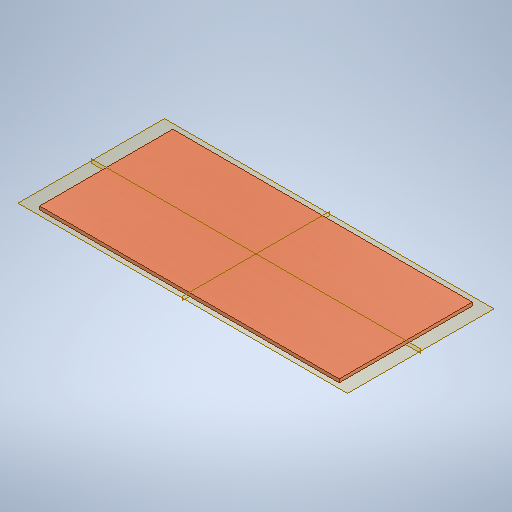
# Autodesk Inventor part: Peça apenas para Exercício
Saved by Autodesk Inventor 2025.2 (Build 292293000, 293)
## iProperties
Created: 2025-04-07
Part Number: Peça apenas para Exercício
Material: Madeira (Nogueira)
Document SubType Name: Modeling
Designer: kenay
Density: 0.55 g/cm^3
Appearance: Nogueira - Natural polido
Author: kenay
Autodesk Inventor part; units mm, degrees
sketch "Esboço1" plane through (0, 0, 0) normal (0, 1, 0) x (-1, 0, 0)
  line L0 (-900, 400) -> (900, 400)
  line L1 (900, 400) -> (900, -400)
  line L2 (900, -400) -> (-900, -400)
  line L3 (-900, -400) -> (-900, 400)
  line L4 (-900, 400) -> (900, -400) construction
  line L5 (900, 400) -> (-900, -400) construction
  point P0 (0, 0)
  dimension "d0" = 1800
  dimension "d1" = 800
  constraints: 12 end point, 2 midpoint, 2 parallel, 1 horizontal, 1 perpendicular
  measures "d0" distance of L1.end L2.end
  measures "d1" distance of L0.end L1.end
extrude "Extrusão1" add sketch "Esboço1" along normal mid plane 20
